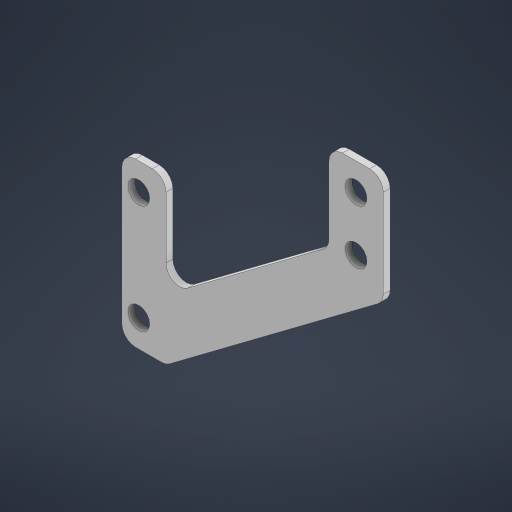
# Autodesk Inventor part: funnelPoly
Saved by Autodesk Inventor 2023.4 (Build 274418000, 418)
## iProperties
Created: 2024-03-08
Part Number: funnelPoly
Material: Generic
Document SubType Name: Modeling
Designer: Meer
Density: 1 g/cm^3
Appearance: Default
Author: Meer
Autodesk Inventor part; units mm, degrees
ref_plane "YZ Plane" through (0, 0, 0) normal (1, 0, 0) x (0, 1, 0)
ref_plane "XZ Plane" through (0, 0, 0) normal (0, 1, 0) x (-1, 0, 0)
ref_plane "XY Plane" through (0, 0, 0) normal (0, 0, 1) x (1, 0, 0)
sketch "Sketch1" plane through (0, 0, 0) normal (0, 0, 1) x (1, 0, 0)
  circle A0 centre (50.8, 50.8) radius 2.54
  circle A1 centre (50.8, 38.1) radius 2.54
  line L0 (50.8, 57.15) -> (57.15, 57.15)
  line L1 (57.15, 57.15) -> (57.15, 50.8)
  line L2 (50.8, 57.15) -> (44.45, 57.15)
  line L3 (44.45, 57.15) -> (44.45, 31.75)
  line L4 (44.45, 31.75) -> (57.15, 31.75)
  circle A2 centre (0, 0) radius 2.54
  circle A3 centre (0, 25.4) radius 2.54
  line L5 (57.15, 50.8) -> (57.15, 31.75)
  line L6 (50.8, 38.1) -> (50.8, 44.45)
  line L7 (50.8, 38.1) -> (57.15, 31.75)
  line L8 (50.8, 38.1) -> (44.45, 44.45)
  line L9 (0, 0) -> (6.35, 0)
  line L10 (6.35, 0) -> (6.35, 31.75)
  line L11 (6.35, -6.35) -> (6.35, 0)
  line L12 (0, 0) -> (6.35, -6.35)
  line L13 (0, 25.4) -> (0, 31.75)
  line L14 (0, 31.75) -> (-3.9624, 31.75)
  line L15 (-3.9624, 31.75) -> (-3.9624, -6.35)
  line L16 (-3.9624, -6.35) -> (6.35, -6.35)
  line L17 (6.35, -6.35) -> (57.15, 31.75)
  line L18 (0, 0) -> (-6.358, 6.358)
  line L19 (49.0039, 39.8961) -> (-1.7961, 1.7961)
  line L20 (0, 31.75) -> (6.35, 31.75)
  point P0 (6.35, 7.9056)
  point P1 (44.45, 36.4806)
  dimension "d5" = 5.08
  dimension "d13" = 5.08
  dimension "d3" = 5.08
  dimension "d7" = 6.35
  dimension "d8" = 6.35
  dimension "d12" = 25.4
  dimension "d18" = 5.08
  dimension "d24" = 6.35
  dimension "d29" = 3.9624
  dimension "d30" = 8.9916
  constraints: 42 end point, 6 perpendicular, 3 point on line, 2 centre point, 2 parallel, 2 vertical, 1 horizontal, 1 midpoint, 6 other
  measures "d3" diameter of A0
  measures "d7" distance of L0.start L0.end
  measures "d8" distance of L0.end L1.end
  measures "d12" distance of L2.end L3.end
  measures "d18" diameter of A3
  measures "d24" distance of L6.start L6.end
  measures "d29" distance of L13.end L14.end
  measures "d30" distance of L9.start L18.end
extrude "Extrusion1" add sketch "Sketch1" along normal blind 1.5875 contours A1 L8 L3 L2 L0 L1 L5 L7 | L7 L4 L3 L19 A1 | L19 L3 L8 | L17 L11 L10 L19 L3 L4 | L12 A2 L9 L11 | L16 L15 L18 A2 L12 | L19 A2 L18 L15 L14 L20 L10 | L10 L9 A2 L19
fillet "Fillet1" radius 3.175 9 edges at (44.45, 57.15, 0.7937) (57.15, 57.15, 0.7937) (57.15, 31.75, 0.7937) (44.45, 36.4806, 0.7937) (6.35, 7.9056, 0.7937) (6.35, 31.75, 0.7937) (-3.9624, 31.75, 0.7937) (-3.9624, -6.35, 0.7937) (6.35, -6.35, 0.7937)
body "Solid1"
